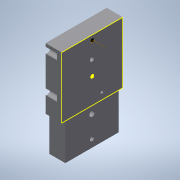
# Autodesk Inventor part: mounting base
Saved by Autodesk Inventor 2020 (Build 240168000, 168)
## iProperties
Created: 2015-12-01
Part Number: mounting base
Material: Generic
Document SubType Name: Modeling
Designer: physics
Density: 1 g/cm^3
Appearance: Default
Author: physics
Autodesk Inventor part; units mm, degrees
ref_plane "YZ Plane" through (0, 0, 0) normal (1, 0, 0) x (0, 1, 0)
ref_plane "XZ Plane" through (0, 0, 0) normal (0, 1, 0) x (-1, 0, 0)
ref_plane "XY Plane" through (0, 0, 0) normal (0, 0, 1) x (1, 0, 0)
sketch "Sketch1" plane through (0, 0, 0) normal (1, 0, 0) x (0, 1, 0)
  line L0 (0, 0) -> (50.8, 0)
  line L1 (50.8, 0) -> (50.8, -50.8)
  line L2 (50.8, -50.8) -> (0, -50.8)
  line L3 (0, -50.8) -> (0, 0)
  circle A0 centre (46.9392, -25.4) radius 0.889
  circle A1 centre (20.955, -25.4) radius 1.27
  line L4 (20.955, -25.4) -> (20.955, -50.8) construction
  line L5 (46.9392, -25.4) -> (46.9392, -50.8) construction
  line L6 (20.955, -25.4) -> (50.8, -25.4) construction
  line L7 (46.9392, -25.4) -> (50.8, -25.4) construction
  dimension "d0" = 50.8
  dimension "d2" = 50.8
  dimension "d3" = 25.4
  dimension "d4" = 25.4
  dimension "d5" = 29.845
  dimension "d6" = 3.8608
  dimension "d7" = 2.54
  dimension "d8" = 1.778
  constraints: 16 end point, 4 perpendicular, 2 centre point, 2 midpoint, 2 parallel, 2 point on line, 1 horizontal
  measures "d0" distance of L0.end L1.end
  measures "d2" distance of L1.end L2.end
  measures "d3" distance of L4.start L4.end
  measures "d4" distance of L5.start L5.end
  measures "d5" distance of L4.start L6.end
  measures "d6" distance of L5.start L7.end
  measures "d7" diameter of A1
  measures "d8" diameter of A0
extrude "Extrusion1" add sketch "Sketch1" along normal blind 12.7
sketch "Sketch2" plane through (0, 0, -50.8) normal (0, -1, 0) x (1, 0, 0)
  line L0 (0, 0) -> (12.7, 0) projected
  line L1 (0, 50.8) -> (12.7, 50.8) projected
  line L2 (6.35, 50.8) -> (6.35, 40.4) construction
  line L3 (6.35, 0) -> (6.35, 10.4) construction
  circle A0 centre (6.35, 10.4) radius 3.175
  circle A1 centre (6.35, 40.4) radius 3.175
  line L4 (12.7, 50.8) -> (12.7, 0) projected
  line L5 (6.35, 40.4) -> (6.35, 10.4) construction
  dimension "d14" = 6.35
  dimension "d15" = 6.35
  dimension "d77" = 30
  constraints: 6 end point, 2 centre point, 2 coincident, 2 collinear, 2 midpoint, 1 parallel, 1 perpendicular
  measures "d14" diameter of A0
  measures "d15" diameter of A1
  measures "d77" distance of L5.start L5.end
extrude "Extrusion2" [suppressed]
sketch "Sketch4" plane through (0, 0, 0) normal (-1, 0, 0) x (0, 0, 1)
  line L0 (0, 0) -> (0, 50.8) projected
  line L1 (0, 50.8) -> (0, 45.72) construction
  line L2 (0, 45.72) -> (-1.27, 45.72) construction
  circle A0 centre (-1.27, 45.72) radius 2.794
  line L3 (-1.27, 45.72) -> (-1.27, 15.8242) construction
  circle A1 centre (-1.27, 15.8242) radius 2.794
  dimension "d23" = 5.08
  dimension "d24" = 1.27
  dimension "d25" = 5.588
  dimension "d26" = 29.8958
  dimension "d27" = 5.588
  constraints: 6 end point, 2 centre point, 2 coincident, 2 perpendicular, 1 point on line
  measures "d23" distance of L0.end L1.end
  measures "d24" distance of L1.end L2.end
  measures "d25" diameter of A0
  measures "d26" distance of L3.start L3.end
  measures "d27" diameter of A1
extrude "Extrusion4" cut sketch "Sketch4" against normal blind 6.604
sketch "Sketch5" plane through (0, 0, 0) normal (-1, 0, 0) x (0, 0, 1)
  line L0 (0, 48.2087) -> (0, 50.8) projected
  line L1 (0, 50.8) -> (-50.8, 50.8) projected
  line L2 (0, 18.3129) -> (0, 43.2313) projected
  line L3 (-50.8, -12.7) -> (0, -12.7)
  line L4 (0, -12.7) -> (0, 50.8)
  line L5 (0, 50.8) -> (-50.8, 50.8)
  line L6 (-50.8, 50.8) -> (-50.8, -12.7)
  line L7 (-38.1, 4.3981) -> (-38.1, 11.8033)
  line L8 (-38.1, 4.3981) -> (-35.56, 4.3981)
  line L9 (-35.56, 4.3981) -> (-35.56, 6.9381)
  arc A0 (-35.56, 6.9381) -> (-35.56, 11.8033) centre (-34.8292, 9.3707) ccw
  line L10 (-35.56, 11.8033) -> (-38.1, 11.8033)
  line L11 (-45.72, 11.8033) -> (-45.72, 6.7233)
  line L12 (-45.72, 11.8033) -> (-40.64, 11.8033)
  line L13 (-40.64, 11.8033) -> (-40.64, 6.7233)
  circle A1 centre (-43.18, 6.7233) radius 2.54
  line L14 (-50.8, -7.7566) -> (-38.1, -7.7566) construction
  line L15 (-50.8, -3.6438) -> (-45.72, -3.6438) construction
  line L16 (-40.64, 6.7233) -> (-45.72, 6.7233) construction
  line L17 (-45.72, 11.8033) -> (-40.64, 11.8033)
  arc A2 (-40.64, 6.7233) -> (-45.72, 6.7233) centre (-43.18, 6.7233) ccw
  circle A3 centre (-25.4, 20.955) radius 1.27 projected
  circle A4 centre (-43.18, 7.6582) radius 0.935
  line L18 (-42.245, 7.6582) -> (-42.245, 11.8033)
  line L19 (-42.245, 11.8033) -> (-44.115, 11.8033)
  line L20 (-44.115, 11.8033) -> (-44.115, 7.6582)
  line L21 (-44.115, 11.8033) -> (-42.245, 11.8033)
  circle A5 centre (-34.8292, 9.3707) radius 1.27
  line L22 (-50.8, 0) -> (0, 0) projected
  dimension "d46" = 12.7
  dimension "d47" = 5.08
  dimension "d48" = 5.08
  dimension "d49" = 2.54
  dimension "d50" = 2.54
  dimension "d52" = 2.54
  dimension "d53" = 5.08
  dimension "d57" = 58.5566
  dimension "d58" = 54.4438
  dimension "d59" = 35.56
  dimension "d60" = 0
  dimension "d61" = 63.5
  dimension "d62" = 0
  dimension "d64" = 38.1
  dimension "d67" = 1.8699
  dimension "d80" = 11.8033
  dimension "d81" = 4.3981
  dimension "d82" = 11.8033
  constraints: 38 end point, 10 perpendicular, 7 point on circle, 6 point on line, 6 tangent, 5 centre point, 3 parallel, 2 coincident, 1 collinear, 1 equal radius, 1 midpoint
  measures "d46" distance of L14.start L14.end
  measures "d47" distance of L15.start L15.end
  measures "d48" distance of L11.start L12.end
  measures "d49" distance of L10.start L7.end
  measures "d50" radius of A0
  measures "d52" distance of L8.end L9.end
  measures "d53" distance of L11.start L11.end
  measures "d57" distance between parallel lines of L5 L14
  measures "d58" distance between parallel lines of L5 L15
  measures "d59" distance between parallel lines of L4 L9
  measures "d60" distance between parallel lines of L1 L5
  measures "d61" distance between parallel lines of L1 L3
  measures "d62" distance between parallel lines of L0 L4
  measures "d64" distance between parallel lines of L2 L7
  measures "d67" diameter of A4
  measures "d80" distance between parallel lines of L22 L10
  measures "d81" distance between parallel lines of L22 L8
  measures "d82" distance between parallel lines of L22 L12
extrude "Extrusion5" add sketch "Sketch5" along normal blind 2.54 contours L7 L10 A0 L9 L8 | L12 L20 A1 L11 | A1 L20 A4 L18 | L12 L18 A1 L20 | A1 L18 L12 L13 | A1 L18 A4 L20 | A4 | A5
sketch "Sketch6" plane through (-2.54, 0, 0) normal (-1, 0, 0) x (0, 0, 1)
  arc A0 (-35.56, 6.9381) -> (-35.56, 11.8033) centre (-34.8292, 9.3707) ccw projected
  line L0 (-35.56, 11.8033) -> (-38.1, 11.8033) projected
  circle A1 centre (-34.8292, 9.3707) radius 1.27
  line L1 (-35.56, 11.8033) -> (-35.56, 6.9381)
  point P0 (0, 0)
  dimension "d68" = 2.54
  constraints: 2 end point, 1 centre point, 1 coincident, 1 perpendicular
  measures "d68" diameter of A1
extrude "Extrusion6" cut sketch "Sketch6" against normal blind 2.54 contours L1 A1 | A1 L1
sketch "Sketch7" plane through (-2.54, 0, 0) normal (-1, 0, 0) x (0, 0, 1)
  arc A0 (-45.72, 6.7233) -> (-40.64, 6.7233) centre (-43.18, 6.7233) ccw projected
  line L0 (-40.64, 11.8033) -> (-45.72, 11.8033) projected
  line L1 (-44.2316, 11.8033) -> (-42.1284, 11.8033)
  line L2 (-42.1284, 11.8033) -> (-42.1284, 6.7233)
  line L3 (-42.1284, 6.7233) -> (-44.2316, 6.7233)
  line L4 (-44.2316, 6.7233) -> (-44.2316, 11.8033)
  circle A1 centre (-43.18, 6.7233) radius 1.0516
  point P0 (0, 0)
  dimension "d71" = 2.1033
  constraints: 8 end point, 2 parallel, 2 point on circle, 1 centre point, 1 coincident, 1 horizontal, 1 perpendicular, 1 point on line, 1 tangent
  measures "d71" diameter of A1
extrude "Extrusion7" cut sketch "Sketch7" against normal blind 2.54
sketch "Sketch8" plane through (12.7, 0, 0) normal (1, 0, 0) x (0, 0, -1)
  circle A0 centre (25.4, 20.955) radius 1.27 projected
  circle A1 centre (25.4, 46.9392) radius 0.889 projected
  line L0 (0, 50.8) -> (0, 0) projected
  line L1 (0, 0) -> (50.8, 0) projected
  line L2 (0, 50.8) -> (50.8, 50.8)
  line L3 (50.8, 50.8) -> (50.8, 0)
  line L4 (50.8, 0) -> (0, 0)
  line L5 (0, 0) -> (0, 50.8)
  constraints: 8 end point, 2 parallel, 1 horizontal, 1 perpendicular
extrude "Extrusion8" cut sketch "Sketch8" against normal blind 2.4384
sketch "Sketch9" plane through (10.2616, 0, 0) normal (1, 0, 0) x (0, 0, -1)
  circle A0 centre (25.4, 20.955) radius 1.27 projected
  circle A1 centre (25.4, 46.9392) radius 0.889 projected
  line L0 (0, 0) -> (0, 50.8) projected
  line L1 (50.8, 0) -> (0, 0) projected
  line L2 (50.8, 50.8) -> (50.8, 0) projected
  line L3 (0, 50.8) -> (50.8, 50.8) projected
  circle A2 centre (25.4, 46.9392) radius 0.889
  constraints: 1 centre point, 1 coincident, 1 concentric
sketch "Sketch12" plane through (0, 50.8, 0) normal (0, 1, 0) x (1, 0, 0)
  line L0 (10.2616, 0) -> (10.2616, 50.8) projected
  line L1 (10.2616, 15.875) -> (10.2616, 34.925)
  line L2 (10.2616, 34.925) -> (0, 34.925)
  line L3 (0, 34.925) -> (0, 15.875)
  line L4 (0, 15.875) -> (10.2616, 15.875)
  line L5 (10.2616, 15.875) -> (0, 34.925) construction
  line L6 (10.2616, 34.925) -> (0, 15.875) construction
  point P0 (5.1308, 25.4)
  dimension "d84" = 19.05
  constraints: 12 end point, 2 midpoint, 2 parallel, 1 collinear, 1 perpendicular
  measures "d84" distance of L1.start L1.end
extrude "Extrusion9" add sketch "Sketch12" along normal blind 25.4
sketch "Sketch14" plane through (0, 0, 0) normal (-1, 0, 0) x (0, 0, 1)
  line L0 (-44.2316, 6.7233) -> (-44.2316, 11.8033) projected
  line L1 (-22.86, 55.5625) -> (-22.86, 71.4375)
  line L2 (-22.86, 71.4375) -> (-27.94, 71.4375)
  line L3 (-27.94, 71.4375) -> (-27.94, 55.5625)
  line L4 (-27.94, 55.5625) -> (-22.86, 55.5625)
  line L5 (-22.86, 55.5625) -> (-27.94, 71.4375) construction
  line L6 (-22.86, 71.4375) -> (-27.94, 55.5625) construction
  circle A0 centre (-25.4, 71.4375) radius 2.54
  circle A1 centre (-25.4, 55.5625) radius 2.54
  line L7 (-15.875, 50.8) -> (-15.875, 76.2) projected
  point P0 (-25.4, 63.5)
  dimension "d87" = 5.08
  dimension "d88" = 15.875
  dimension "d91" = 9.525
  constraints: 12 end point, 4 midpoint, 3 parallel, 2 horizontal alignment, 1 perpendicular, 4 other
  measures "d87" distance of L2.end L1.end
  measures "d88" distance of L2.end L3.end
  measures "d91" distance from line of L7 point (-25.4, 63.5)
extrude "Extrusion10" cut sketch "Sketch14" against normal blind 25.4
sketch "Sketch15" plane through (0, 0, 0) normal (-1, 0, 0) x (0, 0, 1)
  circle A0 centre (-25.4, 20.955) radius 1.27 projected
  circle A1 centre (-25.4, 20.955) radius 2.54
  dimension "d92" = 5.08
  constraints: 1 centre point, 1 coincident
  measures "d92" diameter of A1
extrude "Extrusion11" cut sketch "Sketch15" against normal blind 6.35
sketch "Sketch16" plane through (10.2616, 0, 0) normal (1, 0, 0) x (0, 0, -1)
  circle A0 centre (25.4, 20.955) radius 1.27 projected
  circle A1 centre (25.4, 46.9392) radius 0.889 projected
  circle A2 centre (33.6553, 5.4225) radius 0.889
  dimension "d99" = 17.59
  dimension "d100" = 1.778
  dimension "d103" = 207.99
  constraints: 1 centre point, 1 coincident
  measures "d99" distance of point (33.655, 5.423) A0.centre
  measures "d100" diameter of A2
extrude "Extrusion12" cut sketch "Sketch16" against normal up to next contours A2
sketch "Sketch17" plane through (0, 0, 0) normal (-1, 0, 0) x (0, 0, 1)
  circle A0 centre (-33.6553, 5.4225) radius 0.889 projected
  circle A1 centre (-25.4, 20.955) radius 2.54 projected
  line L0 (-22.86, 71.4375) -> (-22.86, 55.5625) projected
  arc A2 (-27.94, 55.5625) -> (-22.86, 55.5625) centre (-25.4, 55.5625) ccw projected
  line L1 (-27.94, 55.5625) -> (-27.94, 71.4375) projected
  arc A3 (-22.86, 71.4375) -> (-27.94, 71.4375) centre (-25.4, 71.4375) ccw projected
  line L2 (-45.72, 11.8033) -> (-44.2316, 11.8033) projected
  line L3 (-44.2316, 6.7233) -> (-44.2316, 11.8033) projected
  arc A4 (-44.2316, 6.7233) -> (-42.1284, 6.7233) centre (-43.18, 6.7233) ccw projected
  line L4 (-42.1284, 11.8033) -> (-42.1284, 6.7233) projected
  line L5 (-42.1284, 11.8033) -> (-40.64, 11.8033) projected
  line L6 (-40.64, 11.8033) -> (-40.64, 6.7233) projected
  arc A5 (-45.72, 6.7233) -> (-40.64, 6.7233) centre (-43.18, 6.7233) ccw projected
  line L7 (-45.72, 6.7233) -> (-45.72, 11.8033) projected
  line L8 (-38.1, 11.8033) -> (-35.56, 11.8033) projected
  arc A6 (-35.56, 6.9381) -> (-35.56, 11.8033) centre (-34.8292, 9.3707) ccw projected
  line L9 (-35.56, 6.9381) -> (-35.56, 4.3981) projected
  line L10 (-35.56, 4.3981) -> (-38.1, 4.3981) projected
  line L11 (-38.1, 4.3981) -> (-38.1, 11.8033) projected
  arc A7 (0, 48.2087) -> (0, 43.2313) centre (-1.27, 45.72) ccw projected
  line L12 (0, 50.8) -> (-15.875, 50.8) projected
  line L13 (-34.925, 50.8) -> (-34.925, 76.2) projected
  line L14 (-34.925, 50.8) -> (-50.8, 50.8) projected
  line L15 (-50.8, 50.8) -> (-50.8, 0) projected
  line L16 (-50.8, 0) -> (0, 0) projected
  line L17 (0, 0) -> (0, 13.3355) projected
  arc A8 (0, 18.3129) -> (0, 13.3355) centre (-1.27, 15.8242) ccw projected
  circle A9 centre (-25.4, 46.9392) radius 0.889 projected
  line L18 (-34.925, 50.8) -> (-34.925, 76.2)
  line L19 (-15.875, 76.2) -> (-34.925, 76.2)
  line L20 (-15.875, 76.2) -> (-15.875, 50.8)
  line L21 (-15.875, 50.8) -> (0, 50.8)
  line L22 (0, 50.8) -> (0, 48.2087)
  arc A10 (0, 48.2087) -> (0, 43.2313) centre (-1.27, 45.72) ccw
  arc A11 (0, 18.3129) -> (0, 13.3355) centre (-1.27, 15.8242) ccw
  line L23 (0, 43.2313) -> (0, 18.3129)
  line L24 (0, 13.3355) -> (0, 0)
  line L25 (0, 0) -> (-50.8, 0)
  line L26 (-50.8, 0) -> (-50.8, 50.8)
  line L27 (-50.8, 50.8) -> (-34.925, 50.8)
  circle A12 centre (-25.4, 46.9392) radius 0.889
  circle A13 centre (-25.4, 20.955) radius 2.54
  circle A14 centre (-25.4, 33.1527) radius 1.7272
  dimension "d104" = 3.4544
  constraints: 20 end point, 7 collinear, 5 centre point, 4 concentric, 4 point on circle, 3 perpendicular, 2 coincident
  measures "d104" diameter of A14
extrude "Extrusion13" add sketch "Sketch17" along normal blind 3
sketch "Sketch18" plane through (0, 33.1527, -25.4) normal (-1, 0, 0) x (0, 0, 1)
  circle A0 centre (0, 0) radius 1.7272 projected
  circle A1 centre (0, 0) radius 1.7272
  point P0 (25.4, -33.1527)
  constraints: 1 centre point, 1 coincident, 1 concentric
extrude "Extrusion14" cut sketch "Sketch18" against normal up to surface (10.2616 mm away)
sketch "Sketch20" plane through (10.2616, 0, 0) normal (1, 0, 0) x (0, 0, -1)
  circle A0 centre (25.4, 33.1527) radius 1.7272 projected
  circle A1 centre (25.4, -6.096) radius 2.2225
  line L0 (0, 0) -> (0, 50.8) projected
  line L1 (50.8, 0) -> (0, 0) projected
  line L2 (3.175, 0) -> (47.625, 0)
  line L3 (47.625, 0) -> (47.625, -30.48)
  line L4 (47.625, -30.48) -> (3.175, -30.48)
  line L5 (3.175, -30.48) -> (3.175, 0)
  dimension "d111" = 4.445
  dimension "d114" = 0
  dimension "d117" = 6.096
  dimension "d118" = 44.45
  dimension "d119" = 30.48
  dimension "d120" = 3.175
  constraints: 8 end point, 2 parallel, 1 centre point, 1 horizontal, 1 perpendicular, 1 point on line
  measures "d111" diameter of A1
  measures "d114" horizontal distance of A1.centre A0.centre
  measures "d117" distance from line of L1 A1.centre
  measures "d118" distance of L3.end L4.end
  measures "d119" distance of L2.end L3.end
  measures "d120" distance between parallel lines of L0 L5
extrude "Extrusion16" add sketch "Sketch20" against normal up to surface (13.2616 mm away) contours L3 L4 L5 L1
sketch "Sketch21" plane through (10.2616, 0, 0) normal (1, 0, 0) x (0, 0, -1)
  line L0 (22.86, 55.5625) -> (22.86, 71.4375) projected
  arc A0 (27.94, 71.4375) -> (22.86, 71.4375) centre (25.4, 71.4375) ccw projected
  line L1 (27.94, 71.4375) -> (27.94, 55.5625) projected
  arc A1 (22.86, 55.5625) -> (27.94, 55.5625) centre (25.4, 55.5625) ccw projected
  line L2 (15.875, 50.8) -> (34.925, 50.8)
  line L3 (34.925, 50.8) -> (34.925, 76.2)
  line L4 (34.925, 76.2) -> (15.875, 76.2)
  line L5 (15.875, 76.2) -> (15.875, 50.8)
  constraints: 8 end point, 2 parallel, 1 horizontal, 1 perpendicular
extrude "Extrusion17" cut sketch "Sketch21" against normal up to surface (13.2616 mm away)
sketch "Sketch22" plane through (0, 9.3707, -34.8292) normal (-1, 0, 0) x (0, 0, 1)
  circle A0 centre (0, 0) radius 1.27 projected
  circle A1 centre (0, 0) radius 1.27
  point P0 (34.8292, -9.3707)
  constraints: 1 centre point, 1 coincident, 1 concentric
extrude "Extrusion18" add sketch "Sketch22" along normal up to surface (3 mm away)
sketch "Sketch23" plane through (10.2616, 0, 0) normal (1, 0, 0) x (0, 0, -1)
  line L0 (47.625, -30.48) -> (3.175, -30.48) projected
  circle A0 centre (25.4, -24.13) radius 1.7272
  dimension "d127" = 3.4544
  dimension "d128" = 6.35
  constraints: 1 centre point
  measures "d127" diameter of A0
  measures "d128" distance from line of L0 A0.centre
extrude "Extrusion19" cut sketch "Sketch23" against normal up to next
sketch "Sketch24" plane through (-3, 0, 0) normal (-1, 0, 0) x (0, 0, 1)
  circle A0 centre (-25.4, -6.096) radius 2.2225 projected
  circle A1 centre (-25.4, -6.096) radius 3.425
  point P0 (0, 0)
  dimension "d131" = 6.85
  constraints: 1 centre point, 1 coincident
  measures "d131" diameter of A1
extrude "Extrusion20" cut sketch "Sketch24" against normal blind 4.2
thicken "Thicken1" operation add thickness 0.175 both sides no extend neighbours yes toward (0, -0.0804666, 0.9967573) faces at (-0.2, -6.3716, -21.9861)
sketch "Sketch26" plane through (6.35, 20.955, -25.4) normal (-1, 0, 0) x (0, 0, 1)
  circle A0 centre (0, 0) radius 1.1303
  circle A1 centre (0, 0) radius 1.27
  point P0 (25.4, -20.955)
  dimension "d159" = 2.2606
  constraints: 2 centre point, 1 coincident
  measures "d159" diameter of A0
extrude "Extrusion23" add sketch "Sketch26" against normal blind 3.912
sketch "Sketch27" plane through (10.2616, 0, 0) normal (1, 0, 0) x (0, 0, -1)
  circle A0 centre (25.4, 46.9392) radius 0.889 projected
  circle A1 centre (25.4, 46.9392) radius 1.1303
  circle A2 centre (33.6553, 5.4225) radius 0.889 projected
  circle A3 centre (33.6553, 5.4225) radius 1.1303
  point P0 (0, 0)
  dimension "d162" = 2.2606
  dimension "d163" = 2.2606
  constraints: 2 centre point, 2 coincident
  measures "d162" diameter of A1
  measures "d163" diameter of A3
extrude "Extrusion24" cut sketch "Sketch27" against normal blind 10 contours A0 | A1 | A2 | A3
sketch "Sketch28" plane through (-3, 0, 0) normal (-1, 0, 0) x (0, 0, 1)
  circle A0 centre (-33.6553, 5.4225) radius 1.1303 projected
  circle A1 centre (-33.6553, 5.4225) radius 2.325
  circle A2 centre (-25.4, 46.9392) radius 0.889 projected
  circle A3 centre (-25.4, 46.9392) radius 2.325
  point P0 (0, 0)
  dimension "d166" = 4.65
  dimension "d167" = 4.65
  constraints: 2 centre point, 2 coincident
  measures "d166" diameter of A1
  measures "d167" diameter of A3
extrude "Extrusion25" cut sketch "Sketch28" against normal blind 3.5
sketch "Sketch29" plane through (-3, 0, 0) normal (-1, 0, 0) x (0, 0, 1)
  circle A0 centre (-33.6553, 5.4225) radius 0.889 projected
  circle A1 centre (-33.6553, 5.4225) radius 1.1303
  circle A2 centre (-25.4, 46.9392) radius 1.1303 projected
  circle A3 centre (-25.4, 46.9392) radius 1.1303
  point P0 (0, 0)
  dimension "d170" = 2.2606
  dimension "d171" = 2.2606
  constraints: 2 centre point, 2 coincident
  measures "d170" diameter of A1
  measures "d171" diameter of A3
extrude "Extrusion26" cut sketch "Sketch29" against normal blind 10 contours A0 | A1 | A2
body "Solid1"
